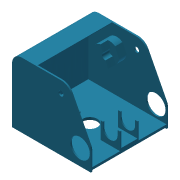
# Autodesk Inventor part: Base
Saved by Autodesk Inventor 2016 (Build 200138000, 138)
## iProperties
Created: 2015-05-18
Part Number: Base
Material: Aluminum 6061
Document SubType Name: Modeling
Designer: CHUNGBK
Density: 2.7 g/cm^3
Appearance: Turquoise
Author: CHUNGBK
Autodesk Inventor part; units mm, degrees
ref_plane "YZ Plane" through (0, 0, 0) normal (1, 0, 0) x (0, 1, 0)
ref_plane "XZ Plane" through (0, 0, 0) normal (0, 1, 0) x (-1, 0, 0)
sketch "Sketch1" plane through (0, 0, 0) normal (0, 1, 0) x (-1, 0, 0)
  line L0 (0, 0) -> (205.5813, 0)
  line L1 (205.5813, 0) -> (205.5813, -193.675)
  line L2 (205.5813, -193.675) -> (0, -193.675)
  line L3 (0, -193.675) -> (0, 0)
  dimension "d0" = 193.675
  dimension "d1" = 205.5813
  constraints: 8 end point, 2 parallel, 1 horizontal, 1 perpendicular
  measures "d0" distance of L2.end L0.start
  measures "d1" distance of L1.end L2.end
extrude "Extrusion1" add sketch "Sketch1" along normal blind 6.35
sketch "Sketch2" plane through (-205.5813, 0, 0) normal (0, 0, 1) x (1, 0, 0)
  line L0 (205.5813, -3.9687) -> (0, -3.9688)
  line L1 (0, -3.9688) -> (0, 140.4938)
  line L2 (25.4, 165.8937) -> (127.6349, 165.8937)
  line L3 (205.5813, 43.8638) -> (205.5813, -3.9687)
  line L4 (0, 0) -> (0, 6.35) projected
  line L5 (0, 0) -> (205.5813, 0) projected
  arc A0 (25.4, 165.8937) -> (0, 140.4938) centre (25.4, 140.4938) ccw
  line L6 (205.5813, 0) -> (205.5813, 6.35) projected
  line L7 (202.7746, 55.47) -> (154.4645, 149.5136)
  arc A1 (154.4645, 149.5136) -> (127.6349, 165.8937) centre (127.6349, 135.7313) ccw
  arc A2 (205.5813, 43.8638) -> (202.7746, 55.47) centre (180.1813, 43.8638) ccw
  circle A3 centre (127.6349, 135.7313) radius 6.35
  circle A4 centre (177.6413, 37.3062) radius 25.4
  line L8 (203.0413, 37.3063) -> (203.0413, -3.9687) construction
  line L9 (177.6413, 11.9062) -> (205.5813, 11.9063) construction
  point P0 (205.5813, 50.0063)
  point P1 (146.05, 165.8938)
  dimension "d4" = 3.9688
  dimension "d6" = 25.4
  dimension "d7" = 169.8625
  dimension "d8" = 146.05
  dimension "d9" = 53.975
  dimension "d10" = 30.1625
  dimension "d11" = 25.4
  dimension "d12" = 12.7
  dimension "d13" = 50.8
  dimension "d14" = 2.54
  dimension "d15" = 15.875
  constraints: 14 end point, 8 point on circle, 8 tangent, 6 point on line, 5 centre point, 3 perpendicular, 2 collinear, 2 parallel, 1 coincident, 1 horizontal
  measures "d4" distance between parallel lines of L5 L0
  measures "d6" radius of A0
  measures "d7" distance between parallel lines of L2 L0
  measures "d8" distance from line of point (146.05, 165.894) L1
  measures "d9" distance from line of L0 point (205.581, 50.006)
  measures "d10" radius of A1
  measures "d11" radius of A2
  measures "d12" diameter of A3
  measures "d13" diameter of A4
  measures "d14" distance between parallel lines of L3 L8
  measures "d15" distance between parallel lines of L0 L9
extrude "Extrusion2" add sketch "Sketch2" along normal blind 3.81
ref_plane "Work Plane1" through (-205.5813, 0, -96.8375) normal (0, 0, -1) x (-1, 0, 0)
mirror "Mirror1" about plane through (-205.5813, 0, -96.8375) normal (0, 0, -1) of "Extrusion2"
sketch "Sketch3" plane through (-205.5813, 0, 0) normal (0, 0, -1) x (-1, 0, 0)
  line L0 (0, 6.35) -> (-205.5813, 6.35) projected
  line L1 (-1.5875, 6.35) -> (-1.5875, 140.4938)
  arc A0 (0, 140.4938) -> (-25.4, 165.8937) centre (-25.4, 140.4938) ccw projected
  arc A1 (-1.5875, 140.4938) -> (-25.4, 164.3062) centre (-25.4, 140.4938) ccw
  line L2 (-25.4, 164.3062) -> (-63.5, 164.3062)
  line L3 (-63.5, 164.3062) -> (-63.5, 165.8937)
  line L4 (-63.5, 165.8937) -> (-25.4, 165.8937)
  line L5 (0, 140.4938) -> (0, -3.9688) projected
  point P0 (-205.5813, 0)
  dimension "d19" = 1.5875
  dimension "d20" = 1.5875
  dimension "d21" = 63.5
  constraints: 8 end point, 2 perpendicular, 2 point on circle, 1 centre point, 1 coincident, 1 horizontal, 1 point on line, 1 tangent, 1 vertical
  measures "d19" distance between parallel lines of L5 L1
  measures "d20" distance between parallel lines of L4 L2
  measures "d21" distance between parallel lines of L5 L3
extrude "Extrusion3" add sketch "Sketch3" along normal up to surface (193.675 mm away)
sketch "Sketch4" plane through (0, 6.35, 0) normal (1, 0, 0) x (0, 0, -1)
  line L0 (193.675, -6.35) -> (0, -6.35) projected
  line L1 (193.675, -6.35) -> (193.675, -10.3187) projected
  line L2 (193.675, -10.3187) -> (197.485, -10.3187) projected
  line L3 (197.485, -10.3187) -> (197.485, 37.5138) projected
  line L4 (193.675, 37.5138) -> (197.485, 37.5138) projected
  line L5 (193.675, 37.5138) -> (193.675, 0) projected
  line L6 (0, 0) -> (193.675, 0) projected
  line L7 (0, 37.5138) -> (0, 0) projected
  line L8 (0, 37.5138) -> (-3.81, 37.5138) projected
  line L9 (-3.81, -10.3187) -> (-3.81, 37.5138) projected
  line L10 (0, -10.3187) -> (-3.81, -10.3187) projected
  line L11 (0, -6.35) -> (0, -10.3187) projected
  line L12 (121.285, 0) -> (121.285, 44.45)
  line L13 (121.285, 44.45) -> (118.11, 44.45)
  line L14 (118.11, 44.45) -> (118.11, 5.5563)
  line L15 (118.11, 5.5563) -> (75.565, 5.5562)
  line L16 (75.565, 5.5562) -> (75.565, 44.45)
  line L17 (75.565, 44.45) -> (72.39, 44.45)
  line L18 (72.39, 44.45) -> (72.39, 0)
  line L19 (121.285, 0) -> (72.39, 0)
  line L20 (96.8375, -6.35) -> (96.8375, -30.2285) construction
  dimension "d24" = 76.2
  dimension "d25" = 3.175
  dimension "d26" = 5.5563
  dimension "d30" = 44.45
  constraints: 18 end point, 5 perpendicular, 4 point on line, 2 vertical, 1 collinear, 1 midpoint, 2 other
  measures "d24" distance between parallel lines of L3 L12
  measures "d25" distance between parallel lines of L12 L14
  measures "d26" distance between parallel lines of L19 L15
  measures "d30" distance between parallel lines of L6 L17
extrude "Extrusion4" add sketch "Sketch4" against normal blind 50.8 contours L6 L18 L17 L16 L15 L14 L13 L12
sketch "Sketch5" plane through (0, 6.35, -121.285) normal (0, 0, -1) x (-1, 0, 0)
  line L0 (0, 44.45) -> (0, 5.5563) projected
  line L1 (0, 44.45) -> (50.8, 44.45) projected
  line L2 (50.8, 5.5563) -> (50.8, 44.45) projected
  line L3 (0, 5.5563) -> (50.8, 5.5563) projected
  line L4 (25.4, 44.45) -> (25.4, 31.75)
  circle A0 centre (25.4, 31.75) radius 19.05
  line L5 (6.35, 31.75) -> (6.35, 44.45)
  line L6 (44.45, 31.75) -> (44.45, 44.45)
  line L7 (44.45, 44.45) -> (6.35, 44.45)
  point P0 (0, -6.35)
  dimension "d29" = 38.1
  dimension "d31" = 12.7
  constraints: 8 end point, 2 perpendicular, 2 point on circle, 2 point on line, 1 centre point, 1 coincident, 1 collinear, 1 midpoint, 1 vertical
  measures "d29" diameter of A0
  measures "d31" distance of L4.start L4.end
extrude "Extrusion5" cut sketch "Sketch5" against normal blind 50.8 contours L1 A0 L5 | A0 L1 | L1 A0 | L1 L6 A0
sketch "Sketch6" plane through (0, 6.35, 0) normal (0, 1, 0) x (1, 0, 0)
  line L0 (-50.8, 121.285) -> (0, 121.285) projected
  line L1 (0, 121.285) -> (0, 193.675) projected
  line L2 (0, 193.675) -> (-203.9938, 193.675) projected
  line L3 (-203.9938, 193.675) -> (-203.9938, 0) projected
  line L4 (-203.9938, 0) -> (0, 0) projected
  line L5 (0, 0) -> (0, 72.39) projected
  line L6 (0, 72.39) -> (-50.8, 72.39) projected
  line L7 (-50.8, 72.39) -> (-50.8, 121.285) projected
  line L8 (-205.5813, 0) -> (0, 193.675)
  circle A0 centre (-102.7906, 96.8375) radius 19.05
  point P0 (-205.5813, 0)
  dimension "d36" = 38.1
  constraints: 2 end point, 1 centre point, 1 coincident, 1 midpoint
  measures "d36" diameter of A0
extrude "Extrusion7" cut sketch "Sketch6" against normal through all contours A0 L8 | L8 A0
sketch "Sketch7" plane through (-205.5813, 0, 3.81) normal (0, 0, 1) x (1, 0, 0)
  line L0 (0, -3.9688) -> (205.5813, -3.9687) projected
  line L1 (0, 140.4938) -> (0, -3.9688) projected
  line L2 (117.475, 97.6313) -> (106.3625, 64.2938)
  point P0 (205.5813, 0)
  point P1 (111.9187, 80.9625)
  dimension "d39" = 101.6
  dimension "d40" = 117.475
  dimension "d41" = 106.3625
  dimension "d42" = 68.2625
  constraints: 2 end point, 1 midpoint
  measures "d39" distance from line of L0 L2.start
  measures "d40" distance from line of L1 L2.start
  measures "d41" distance from line of L2.end L1
  measures "d42" distance from line of L2.end L0
sketch "Sketch8" plane through (0, -3.9687, -197.485) normal (0, 0, -1) x (-1, 0, 0)
  line L0 (205.5813, 144.4625) -> (205.5813, 0) projected
  line L1 (205.5813, 0) -> (0, 0) projected
  line L2 (113.5063, 125.4125) -> (146.05, 110.7324)
  point P0 (0, 3.9687)
  point P1 (129.7781, 118.0724)
  dimension "d43" = 92.075
  dimension "d44" = 125.4125
  dimension "d45" = 110.7324
  dimension "d46" = 59.5312
  constraints: 2 end point, 1 midpoint
  measures "d43" distance from line of L0 L2.start
  measures "d44" distance from line of L1 L2.start
  measures "d45" distance from line of L1 L2.end
  measures "d46" distance from line of L0 L2.end
sketch "Sketch9" plane through (0, 6.35, 0) normal (0, 1, 0) x (1, 0, 0)
  circle A0 centre (-102.7906, 96.8375) radius 19.05 projected
  line L0 (0, 0) -> (-205.5813, 0) projected
  line L1 (-205.5813, 0) -> (-205.5813, 193.675) projected
  line L2 (-205.5813, 193.675) -> (0, 193.675) projected
  line L3 (0, 193.675) -> (0, 0) projected
  point P0 (-169.7673, 96.8375)
  dimension "d47" = 35.814
  measures "d47" distance from line of L1 point (-169.767, 96.837)
sketch "Sketch10" plane through (0, 6.35, 0) normal (0, 1, 0) x (1, 0, 0)
  circle A0 centre (-169.7673, 96.8375) radius 3.81
  point P0 (0, 0)
  dimension "d48" = 7.62
  constraints: 1 centre point, 1 coincident
  measures "d48" diameter of A0
extrude "Extrusion8" cut sketch "Sketch10" against normal blind 12.7
sketch "Sketch11" plane through (-205.5813, 0, 0) normal (0, 0, -1) x (-1, 0, 0)
  circle A0 centre (-111.9187, 80.9625) radius 25.4
  point P0 (-205.5813, 0)
  dimension "d51" = 50.8
  constraints: 1 centre point, 1 coincident
  measures "d51" diameter of A0
extrude "Extrusion9" add sketch "Sketch11" along normal blind 38.1
sketch "Sketch12" plane through (0, 6.35, -193.675) normal (0, 0, 1) x (1, 0, 0)
  circle A0 centre (-129.7781, 107.7537) radius 25.4
  point P0 (0, -6.35)
  dimension "d54" = 50.8
  constraints: 1 centre point, 1 coincident
  measures "d54" diameter of A0
extrude "Extrusion10" add sketch "Sketch12" along normal blind 38.1
sketch "Sketch14" plane through (-205.5813, 0, 0) normal (0, 0, -1) x (-1, 0, 0)
  circle A0 centre (-111.9187, 80.9625) radius 25.4 projected
  line L0 (-117.475, 97.6313) -> (-106.3625, 64.2938) projected
  line L1 (-137.2582, 79.2095) -> (-90.5954, 94.7638)
  line L2 (-103.8866, 56.8659) -> (-72.4265, 67.3526) construction
  circle A1 centre (-114.5613, 88.8903) radius 11.6048
  line L3 (-124.7702, 83.3722) -> (-103.0833, 90.6011)
  point P0 (-205.5813, 0)
  dimension "d58" = 31.75
  dimension "d59" = 8.3566
  dimension "d60" = 22.86
  constraints: 6 end point, 5 point on circle, 3 point on line, 1 centre point, 1 coincident, 1 perpendicular, 1 tangent
  measures "d58" distance between parallel lines of L2 L1
  measures "d59" distance of A0.centre point (-114.561, 88.89)
  measures "d60" distance of L3.start L3.end
extrude "Extrusion11" cut sketch "Sketch14" along normal blind 38.1 contours L1 A1 A0 | A1 L0 L1 | L1 A1 | L1 L0 A1 picked at (-132.9928, 82.6187)
extrude "Extrusion13" add sketch "Sketch14" along normal blind 19.05 contours L1 A1 A0 | L1 A1 picked at (-132.9928, 82.6187)
sketch "Sketch15" plane through (0, 6.35, -193.675) normal (0, 0, 1) x (1, 0, 0)
  circle A0 centre (-129.7781, 107.7537) radius 25.4 projected
  line L0 (-113.5062, 115.0938) -> (-146.05, 100.4136) projected
  line L1 (-134.1024, 132.7829) -> (-113.8772, 87.9466)
  line L2 (-152.9315, 97.3094) -> (-166.1131, 126.5311) construction
  circle A1 centre (-122.1607, 111.1898) radius 7.9851
  line L3 (-117.768, 96.572) -> (-127.1678, 117.41)
  point P0 (0, -6.35)
  dimension "d63" = 31.75
  dimension "d64" = 22.86
  dimension "d65" = 8.3566
  constraints: 6 end point, 3 point on circle, 3 point on line, 1 perpendicular, 1 tangent, 3 other
  measures "d63" distance between parallel lines of L1 L2
  measures "d64" distance of L3.start L3.end
  measures "d65" distance of point (-122.161, 111.19) A0.centre
extrude "Extrusion12" cut sketch "Sketch15" along normal blind 38.1 contours A0 L1 A1 | A1 L0 L1 | L1 L0 A1 | L1 A1 L0 | L0 A1 L1 picked at (-129.1797, 128.0803)
extrude "Extrusion14" add sketch "Sketch15" along normal blind 19.05 contours A0 L1 A1 | A1 L0 L1 | L1 L0 A1 | L1 A1 L0 | L0 A1 L1 picked at (-129.1797, 128.0803)
sketch "Sketch16" plane through (0, 6.35, -174.625) normal (0, 0, 1) x (1, 0, 0)
  circle A0 centre (-129.7781, 107.7537) radius 25.4 projected
  line L0 (-113.8772, 87.9466) -> (-120.8117, 103.3195) projected
  arc A1 (-127.1678, 117.41) -> (-120.8117, 103.3195) centre (-122.1607, 111.1898) ccw projected
  line L1 (-127.1678, 117.41) -> (-134.1024, 132.7829) projected
  arc A2 (-134.1024, 132.7829) -> (-113.8772, 87.9466) centre (-129.7781, 107.7537) ccw projected
  line L2 (-114.9488, 128.3753) -> (-104.5046, 105.222)
  point P0 (0, -6.35)
  dimension "d72" = 25.4
  constraints: 2 end point, 2 point on circle, 1 parallel
  measures "d72" distance of L2.end L2.start
extrude "Extrusion15" cut sketch "Sketch16" against normal up to surface (19.05 mm away) contours A0 L2
sketch "Sketch17" plane through (-205.5813, 0, -19.05) normal (0, 0, -1) x (-1, 0, 0)
  line L0 (-90.5954, 94.7638) -> (-103.0833, 90.6011) projected
  arc A0 (-124.7702, 83.3722) -> (-103.0833, 90.6011) centre (-114.5613, 88.8903) ccw projected
  line L1 (-124.7702, 83.3722) -> (-137.2582, 79.2095) projected
  arc A1 (-137.2582, 79.2095) -> (-90.5954, 94.7638) centre (-111.9187, 80.9625) ccw projected
  line L2 (-124.7702, 83.3722) -> (-137.2582, 79.2095) projected
  line L3 (-124.7702, 83.3722) -> (-103.0833, 90.6011) projected
  line L4 (-90.5954, 94.7638) -> (-103.0833, 90.6011) projected
  arc A2 (-90.5954, 94.7638) -> (-137.2582, 79.2095) centre (-111.9187, 80.9625) ccw projected
  line L5 (-130.9231, 97.8146) -> (-106.8265, 105.8468)
  point P0 (-205.5813, 0)
  dimension "d75" = 25.4
  constraints: 2 end point, 2 point on circle, 1 parallel
  measures "d75" distance of L5.start L5.end
extrude "Extrusion16" cut sketch "Sketch17" against normal up to surface (19.05 mm away) contours L5 A2
body "Solid1"
